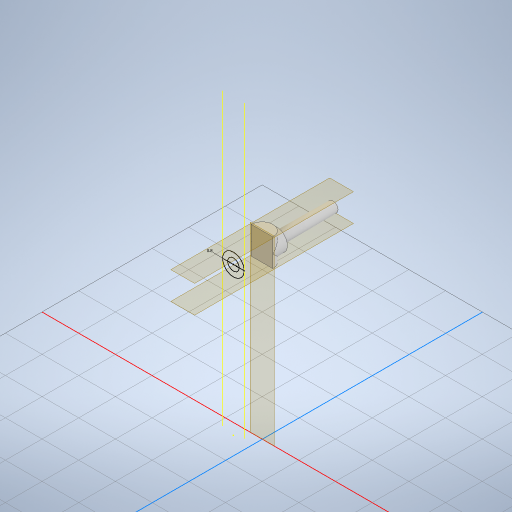
# Autodesk Inventor part: Tube Rotator rod
Saved by Autodesk Inventor 2023 (Build 270158000, 158)
## iProperties
Created: 2023-02-25
Part Number: Tube Rotator rod
Material: Generic
Document SubType Name: Modeling
Designer: James
Density: 1 g/cm^3
Appearance: Default
Author: James
Autodesk Inventor part; units mm, degrees
ref_plane "YZ Plane" through (0, 0, 0) normal (1, 0, 0) x (0, 1, 0)
sketch "Sketch1" plane through (0, 0, 0) normal (0, 1, 0) x (-1, 0, 0)
  circle A0 centre (0, 0) radius 7.5
  dimension "d0" = 15
  constraints: 1 centre point, 1 coincident
  measures "d0" diameter of A0
extrude "Extrusion1" add sketch "Sketch1" along normal blind 205
sketch "Sketch2" plane through (0, 205, 0) normal (0, 1, 0) x (1, 0, 0)
  circle A0 centre (0, 0) radius 3.75
  dimension "d3" = 7.5
  constraints: 1 centre point, 1 coincident
  measures "d3" diameter of A0
ref_plane "Work Plane1" through (0, 0, 20) normal (0, 0, 1) x (1, 0, 0)
extrude "Extrusion2" cut sketch "Sketch2" against normal blind 17
sketch "Sketch3" plane through (0, 0, 20) normal (0, 0, 1) x (1, 0, 0)
  circle A0 centre (0, 199.45) radius 1.75
  line L0 (7.5, 205) -> (-7.5, 205) projected
  circle A1 centre (0, 199.45) radius 2.75
  line L1 (1.6021, 202.225) -> (3.2043, 199.45)
  line L2 (3.2043, 199.45) -> (1.6021, 196.675)
  line L3 (1.6021, 196.675) -> (-1.6021, 196.675)
  line L4 (-1.6021, 196.675) -> (-3.2043, 199.45)
  line L5 (-3.2043, 199.45) -> (-1.6021, 202.225)
  line L6 (-1.6021, 202.225) -> (1.6021, 202.225)
  point P0 (0, 0)
  dimension "d7" = 3.5
  dimension "d8" = 5.55
  dimension "d9" = 5.5
  dimension "d10" = 5.55
  constraints: 12 end point, 2 centre point, 2 coincident, 13 other
  measures "d7" diameter of A0
  measures "d8" distance from line of L0 A0.centre
  measures "d9" diameter of A1
  measures "d10" distance between parallel lines of L3 L6
extrude "Extrusion3" cut sketch "Sketch3" against normal blind 40 contours A0
extrude "Extrusion4" cut sketch "Sketch3" against normal blind 14 contours A1
ref_plane "Work Plane2" through (0, 0, -5) normal (0, 0, 1) x (1, 0, 0)
extrude "Extrusion5" cut sketch "Sketch3" against normal blind 14 from surface at -25 contours A0 | A1 | L1 L2 L3 L4 L5 L6
sketch "Sketch4" plane through (0, 0, 0) normal (0, -1, 0) x (1, 0, 0)
  circle A0 centre (0, 0) radius 3.875
  circle A1 centre (0, 0) radius 7.5
  dimension "d18" = 7.75
  constraints: 2 centre point, 2 coincident
  measures "d18" diameter of A0
extrude "Extrusion6" add sketch "Sketch4" along normal blind 9 contours A0
fillet "Fillet1" radius 2 1 edges at (7.5, 0, 0)
fillet "Fillet2" radius 1 1 edges at (-3.875, -9, 0)
sketch "Sketch5" plane through (0, -9, 0) normal (0, -1, 0) x (1, 0, 0)
  line L0 (0, 0) -> (-4.6313, 0)
  line L1 (0, 0) -> (-4.62, -0.3231)
  line L2 (0, 0) -> (-4.62, 0.3231)
  line L3 (0, 0) -> (2.0302, -4.1626)
  line L4 (0, 0) -> (2.5898, -3.8395)
  line L5 (0, 0) -> (2.3157, -4.0108)
  line L6 (0, 0) -> (2.5898, 3.8395)
  line L7 (0, 0) -> (2.0302, 4.1626)
  line L8 (0, 0) -> (2.3157, 4.0108)
  line L9 (-4.62, -0.3231) -> (-4.62, 0.3231)
  line L10 (2.0302, 4.1626) -> (2.5898, 3.8395)
  line L11 (2.5898, -3.8395) -> (2.0302, -4.1626)
  circle A0 centre (0, 0) radius 1.5
  point P0 (0.8388, -1.2436)
  point P1 (0.8388, 1.2436)
  point P2 (0.6576, 1.3482)
  point P3 (-1.4963, 0.1046)
  point P4 (-1.4963, -0.1046)
  point P5 (0.6576, -1.3482)
  dimension "d25" = 4
  dimension "d29" = 360
  dimension "d31" = 3
  constraints: 24 end point, 4 coincident, 1 centre point, 1 horizontal, 1 symmetric about line, 1 vertical, 26 other
  measures "d31" diameter of A0
extrude "Extrusion7" cut sketch "Sketch5" against normal blind 9 contours L1 A0 L0 | L0 A0 L2 | L5 A0 L3 | L4 A0 L5 | L8 A0 L6 | L7 A0 L8 | A0 L1 L9 L0 | L0 L9 L2 A0 | A0 L5 L11 L3 | L4 L11 L5 A0 | A0 L8 L10 L6 | L7 L10 L8 A0
fillet "Fillet3" radius 2 1 edges at (7.5, 205, 0)
sketch "Sketch6" plane through (0, 0, 20) normal (0, 0, 1) x (1, 0, 0)
  line L0 (-7.5, 2) -> (-7.5, 203) projected
  line L1 (7.5, 2) -> (7.5, 203) projected
  line L2 (-7.5, 102.5) -> (7.5, 102.5)
  circle A0 centre (0, 102.5) radius 7.5
  circle A1 centre (0, 102.5) radius 4
  point P0 (0, 0)
  dimension "d35" = 8
  constraints: 3 midpoint, 2 end point, 1 centre point, 1 coincident, 1 horizontal alignment, 2 other
  measures "d35" diameter of A1
extrude "Extrusion8" add sketch "Sketch6" along normal mid plane 20 from surface at -20
extrude "Extrusion10" cut sketch "Sketch5" against normal blind 9 draft -1.5 contours L1 A0 L0 | L3 A0 L1 | L0 A0 L2 | L5 A0 L3 | L6 A0 L4 | L4 A0 L5 | L8 A0 L6 | L2 A0 L7 | L7 A0 L8
ref_plane "Work Plane3" through (0, 10, 0) normal (0, -1, 0) x (1, 0, 0)
ref_plane "Work Plane4" through (0, 102.5, -10) normal (0, 0, -1) x (-1, 0, 0)
sketch "Sketch7" plane through (0, 0, 0) normal (0, 0, 1) x (1, 0, 0)
  circle A0 centre (0, 102.5) radius 4 projected
  point P0 (0, 0)
extrude "Extrusion11" add sketch "Sketch7" along normal mid plane 100 draft -0.5
fillet "Fillet5" radius 1 2 edges at (-3.5637, 102.5, -50) (-3.5637, 102.5, 50)
ref_plane "Work Plane6" through (0, 112.7125, 0) normal (0, 1, 0) x (-1, 0, 0)
ref_plane "Work Plane5" through (0, 93.6625, 0) normal (0, 1, 0) x (-1, 0, 0)
split "Split4" plane through (0, 93.6625, 0) removes the side toward (0, -1, 0)
split "Split5" plane through (0, 112.7125, 0) removes the side toward (0, 1, 0)
split "Split6" plane through (0, 0, 0) removes the side toward (0, 0, 1)
body "Solid1"
